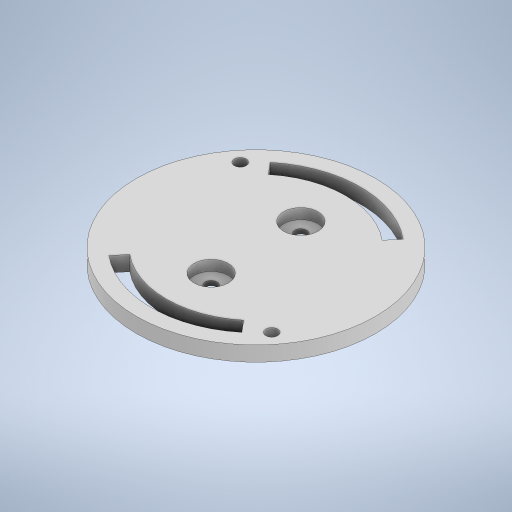
# Autodesk Inventor part: Wrist_Coupling
Saved by Autodesk Inventor 2023 (Build 270158000, 158)
## iProperties
Created: 2023-02-27
Part Number: Wrist_Coupling
Material: Generic
Document SubType Name: Modeling
Designer: adity
Density: 1 g/cm^3
Appearance: Default
Author: adity
Autodesk Inventor part; units mm, degrees
ref_plane "YZ Plane" through (0, 0, 0) normal (1, 0, 0) x (0, 1, 0)
ref_plane "XZ Plane" through (0, 0, 0) normal (0, 1, 0) x (-1, 0, 0)
sketch "Sketch1" plane through (0, 0, 0) normal (0, 1, 0) x (-1, 0, 0)
  circle A0 centre (0, 0) radius 40
  dimension "d0" = 80
  constraints: 1 centre point, 1 coincident
  measures "d0" diameter of A0
sketch "Sketch1 outline for Extrusion1" plane through (0, 0, 0) normal (0, 1, 0) x (-1, 0, 0)
  circle A0 centre (0, 0) radius 40
extrude "Extrusion1" add sketch "Sketch1 outline for Extrusion1" along normal blind 5
sketch "Sketch6" plane through (0, 0, 0) normal (0, -1, 0) x (1, 0, 0)
  line L0 (0, 0) -> (25, 0)
  circle A0 centre (25, 0) radius 10
  line L1 (0, 0) -> (-25, 0)
  line L2 (0, 0) -> (25, 0) construction
  circle A1 centre (-25, 0) radius 10
  dimension "d19" = 25
  dimension "d20" = 20
  dimension "d46" = 25
  dimension "d47" = 180
  dimension "d48" = 20
  constraints: 6 end point, 3 horizontal, 2 centre point, 2 coincident, 1 collinear
  measures "d19" distance of L0.start L0.end
  measures "d20" diameter of A0
  measures "d46" distance of L0.start L1.end
  measures "d47" angle of L1 L2
  measures "d48" diameter of A1
sketch "Sketch6 outline for Extrusion5" plane through (0, 0, 0) normal (0, -1, 0) x (1, 0, 0)
  circle A0 centre (25, 0) radius 10
  circle A1 centre (-25, 0) radius 10
extrude "Extrusion5" cut sketch "Sketch6 outline for Extrusion5" against normal blind 4
sketch "Sketch8" plane through (0, 0, 0) normal (0, -1, 0) x (1, 0, 0)
  circle A0 centre (0, 0) radius 40
  line L0 (21.650635, 27.5) -> (26.777009, 27.5) construction
  line L1 (0, 40) -> (0, 35)
  circle A1 centre (0, 0) radius 35
  line L2 (0, 35) -> (0, 30)
  circle A2 centre (0, 0) radius 30
  line L3 (0, 30) -> (26.457513, 30)
  line L4 (18.027756, 30) -> (15.52731, 25.669099)
  line L5 (18.027756, 30) -> (23.02865, 30) construction
  line L6 (-40, 0) -> (40, 0)
  line L7 (0, -30) -> (0, -40)
  line L8 (0, 30) -> (0, 27)
  line L9 (0, 27) -> (29.512709, 27)
  line L10 (22.271057, 27) -> (27.352779, 27) construction
  line L11 (22.271057, 27) -> (19.056987, 23.169619)
  line L12 (22.271057, 27) -> (27.271264, 27) construction
  line L13 (22.271057, -27) -> (19.056987, -23.169619)
  point P0 (0, -35)
  dimension "d53" = 5
  dimension "d54" = 5
  dimension "d55" = 120
  dimension "d58" = 3
  dimension "d60" = 130
  constraints: 28 end point, 14 point on circle, 6 horizontal, 4 vertical, 2 centre point, 2 coincident, 2 point on line, 2 symmetric about line, 1 equal length, 1 perpendicular, 1 tangent
  measures "d53" distance of L1.start L1.end
  measures "d54" distance of L1.end L2.end
  measures "d55" angle of L4 L5
  measures "d58" distance of L8.start L8.end
  measures "d60" angle of L11 L12
sketch "Sketch8 outline for Extrusion7" plane through (0, 0, 0) normal (0, -1, 0) x (1, 0, 0)
  line L0 (22.271057, -27) -> (19.056987, -23.169619)
  arc A0 (0, -35) -> (22.271057, -27) centre (0, 0) ccw
  line L1 (0, -30) -> (0, -35)
  arc A1 (19.056987, -23.169619) -> (0, -30) centre (0, 0) cw
  line L2 (19.056987, 23.169619) -> (22.271057, 27)
  arc A2 (0, 30) -> (19.056987, 23.169619) centre (0, 0) cw
  line L3 (0, 35) -> (0, 30)
  arc A3 (22.271057, 27) -> (0, 35) centre (0, 0) ccw
extrude "Extrusion7" cut sketch "Sketch8 outline for Extrusion7" against normal up to surface (5 mm away)
ref_plane "Work Plane1" through (0, 0, -32.5) normal (1, 0, 0) x (0, 0, -1)
mirror "Mirror1" about plane through (0, 0, -32.5) normal (1, 0, 0) of "Extrusion7"
sketch "Sketch9" plane through (0, 5, 0) normal (0, 1, 0) x (1, 0, 0)
  circle A0 centre (25, 0) radius 10
  circle A1 centre (-25, 0) radius 10
  arc A2 (-19.056987, -23.169619) -> (19.056987, -23.169619) centre (0, 0) ccw
  line L0 (0, 0) -> (0, -30)
  line L1 (0, 0) -> (0, 30)
  arc A3 (19.056987, 23.169619) -> (-19.056987, 23.169619) centre (0, 0) ccw
  line L2 (0, 0) -> (0, -15)
  circle A4 centre (0, -15) radius 5.75
  line L3 (0, 0) -> (0, 15)
  circle A5 centre (0, 15) radius 5.75
  dimension "d61" = 15
  dimension "d62" = 11.5
  dimension "d63" = 15
  dimension "d64" = 11.5
  constraints: 8 end point, 2 centre point, 2 coincident, 2 midpoint, 2 point on circle, 1 point on line, 1 vertical
  measures "d61" distance of L2.start L2.end
  measures "d62" diameter of A4
  measures "d63" distance of L2.start L3.end
  measures "d64" diameter of A5
sketch "Sketch9 outline for Extrusion8" plane through (0, 5, 0) normal (0, 1, 0) x (1, 0, 0)
  circle A0 centre (0, 15) radius 5.75
  circle A1 centre (0, -15) radius 5.75
extrude "Extrusion8" cut sketch "Sketch9 outline for Extrusion8" against normal blind 3.5
sketch "Sketch10" plane through (0, 1.5, 15) normal (0, 1, 0) x (1, 0, 0)
  circle A0 centre (0, 30) radius 5.75 projected
  circle A1 centre (0, 30) radius 2
  circle A2 centre (0, 0) radius 5.75 projected
  circle A3 centre (0, 0) radius 2
  point P0 (0, 15)
  dimension "d68" = 4
  dimension "d69" = 4
  constraints: 2 centre point, 2 coincident
  measures "d68" diameter of A1
  measures "d69" diameter of A3
sketch "Sketch10 outline for Extrusion9" plane through (0, 1.5, 15) normal (0, 1, 0) x (1, 0, 0)
  circle A0 centre (0, 0) radius 2
  circle A1 centre (0, 30) radius 2
extrude "Extrusion9" cut sketch "Sketch10 outline for Extrusion9" against normal up to surface (1.5 mm away)
sketch "Sketch11" plane through (0, 0, 0) normal (0, -1, 0) x (1, 0, 0)
  line L0 (22.271057, 27) -> (19.056987, 23.169619)
  line L1 (22.271057, 27) -> (22.271057, 22)
  line L2 (22.271057, 22) -> (27.271057, 22)
  circle A0 centre (27.271057, 22) radius 2
  arc A1 (-22.271057, -27) -> (22.271057, -27) centre (0, 0) ccw
  line L3 (-22.271057, -27) -> (-22.271057, -22)
  line L4 (-22.271057, -22) -> (-27.271057, -22)
  circle A2 centre (-27.271057, -22) radius 2
  dimension "d72" = 5
  dimension "d73" = 5
  dimension "d74" = 4
  dimension "d75" = 5
  dimension "d76" = 5
  dimension "d77" = 4
  constraints: 8 end point, 2 centre point, 2 coincident, 2 perpendicular, 2 vertical
  measures "d72" distance of L0.start L1.end
  measures "d73" distance of L1.end L2.end
  measures "d74" diameter of A0
  measures "d75" distance of L3.start L3.end
  measures "d76" distance of L3.end L4.end
  measures "d77" diameter of A2
sketch "Sketch11 outline for Extrusion10" plane through (0, 0, 0) normal (0, -1, 0) x (1, 0, 0)
  circle A0 centre (27.271057, 22) radius 2
  circle A1 centre (-27.271057, -22) radius 2
extrude "Extrusion10" cut sketch "Sketch11 outline for Extrusion10" against normal up to surface (5 mm away)
body "Solid1"
